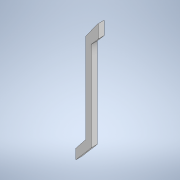
# Autodesk Inventor part: Mannettev2
Saved by Autodesk Inventor 2021 (Build 250183000, 183)
## iProperties
Created: 2020-09-19
Part Number: Mannettev2
Material: Générique
Document SubType Name: Modeling
Designer: Utilisateur
Density: 1 g/cm^3
Appearance: Par défaut
Author: Utilisateur
Autodesk Inventor part; units mm, degrees
ref_plane "YZ Plane" through (0, 0, 0) normal (1, 0, 0) x (0, 1, 0)
ref_plane "XZ Plane" through (0, 0, 0) normal (0, 1, 0) x (-1, 0, 0)
ref_plane "XY Plane" through (0, 0, 0) normal (0, 0, 1) x (1, 0, 0)
sketch "Esquisse1" plane through (0, 0, 0) normal (0, 0, 1) x (1, 0, 0)
  line L0 (15.5804, -42.2686) -> (15.5804, -27.2686)
  line L1 (15.5804, -27.2686) -> (30.5804, -8.3559)
  line L2 (30.5804, -8.3559) -> (30.5804, 126.6441)
  line L3 (48.8358, 151.6441) -> (48.8358, 131.6441)
  line L4 (48.8358, 131.6441) -> (38.5804, 119.6441)
  line L5 (38.5804, 119.6441) -> (38.5804, -15.3559)
  line L6 (38.5804, -15.3559) -> (15.5804, -42.2686)
  line L7 (30.5804, 126.6441) -> (48.8358, 151.6441)
  point P0 (0, 0)
  dimension "d0" = 135
  dimension "d1" = 135
  dimension "d2" = 15
  dimension "d3" = 20
  dimension "d4" = 23
  dimension "d5" = 15
  dimension "d6" = 25
  dimension "d7" = 12
  constraints: 16 end point, 4 parallel, 1 vertical
  measures "d0" distance of L4.end L5.end
  measures "d1" distance of L1.end L2.end
  measures "d2" distance of L0.start L0.end
  measures "d3" distance of L3.start L3.end
  measures "d4" horizontal distance of L5.end L0.start
  measures "d5" horizontal distance of L0.end L1.end
  measures "d6" vertical distance of L2.end L3.start
  measures "d7" vertical distance of L3.end L4.end
extrude "Extrusion1" add sketch "Esquisse1" along normal blind 9
